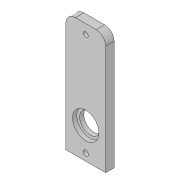
# Autodesk Inventor part: Lidar Sensor Case v4 Piece 1
Saved by Autodesk Inventor 2018.3 (Build 223284000, 284)
## iProperties
Created: 2019-03-27
Part Number: Lidar Sensor Case v4 Piece 1
Material: Generic
Document SubType Name: Modeling
Designer: aye06091
Mass: 10.5036 g
Surface Area: 53.8727 cm^2
Volume: 10.5036 cm^3
Density: 1 g/cm^3
Appearance: Default
Author: aye06091
Autodesk Inventor part; units mm, degrees
ref_plane "YZ Plane" through (0, 0, 0) normal (1, 0, 0) x (0, 1, 0)
ref_plane "XZ Plane" through (0, 0, 0) normal (0, 1, 0) x (-1, 0, 0)
ref_plane "XY Plane" through (0, 0, 0) normal (0, 0, 1) x (1, 0, 0)
sketch "Sketch1" plane through (0, 0, 0) normal (0, 0, 1) x (1, 0, 0)
  line L0 (18.6455, 5.0782) -> (18.6456, 5.0782)
  circle A0 centre (26.2482, -10.4107) radius 8.7948
  line L1 (39.4932, 48.3268) -> (39.4932, -31.0482)
  line L2 (13.0032, -31.0482) -> (13.0032, 48.3268)
  line L3 (13.0032, 48.3268) -> (39.4932, 48.3268)
  line L4 (39.4932, -31.0482) -> (13.0032, -31.0482)
  circle A1 centre (26.2471, -24.96) radius 1.5875
  point P0 (0, 0)
  dimension "d0" = 17.5895
  dimension "d3" = 26.49
  dimension "d4" = 13.245
  dimension "d5" = 58.7375
  dimension "d6" = 79.375
  dimension "d15" = 3.175
  dimension "d25" = 26.49
  dimension "d26" = 13.2461
  constraints: 10 end point, 2 centre point, 2 vertical, 1 horizontal, 1 perpendicular
  measures "d0" diameter of A0
  measures "d3" distance of L2.end L1.start
  measures "d4" distance from line of A0.centre L1
  measures "d5" distance from line of L3 A0.centre
  measures "d6" distance of L1.start L1.end
  measures "d15" diameter of A1
  measures "d25" distance of L1.end L2.start
  measures "d26" distance from line of L1 A1.centre
extrude "Extrusion1" add sketch "Sketch1" against normal blind 5.6134 contours L1 L4 L2 L3 | A1
sketch "Sketch2" plane through (0, 0, 0) normal (0, 0, 1) x (1, 0, 0)
  line L0 (13.0032, 48.3268) -> (39.4932, 48.3268) projected
  circle A0 centre (26.2482, 41.9768) radius 1.6002
  point P0 (0, 0)
  point P1 (0, 0)
  dimension "d10" = 3.2004
  dimension "d12" = 6.35
  constraints: 1 centre point
  measures "d10" diameter of A0
  measures "d12" distance from line of L0 A0.centre
extrude "Extrusion2" cut sketch "Sketch2" against normal blind 5.6134
sketch "Sketch3" plane through (0, 0, 0) normal (0, 0, 1) x (1, 0, 0)
  circle A0 centre (26.2482, -10.4107) radius 8.7947 projected
  circle A1 centre (26.2471, -26.3619) radius 1.7272
  line L0 (39.4932, 48.3268) -> (39.4932, -31.0482) projected
  point P0 (0, 0)
  dimension "d17" = 3.4544
  dimension "d18" = 15.9512
  dimension "d27" = 13.2461
  constraints: 1 centre point
  measures "d17" diameter of A1
  measures "d18" distance of A0.centre A1.centre
  measures "d27" distance from line of L0 A1.centre
extrude "Extrusion3" cut sketch "Sketch3" against normal blind 5.6134 contours A1
fillet "Fillet1" radius 6.35 2 edges at (13.0032, 48.3268, -2.8067) (39.4932, 48.3268, -2.8067)
sketch "Sketch5" plane through (0, 0, -5.6134) normal (0, 0, -1) x (-1, 0, 0)
  circle A0 centre (-26.2482, -10.4107) radius 8.7947 projected
  circle A1 centre (-26.2482, -10.4107) radius 6.9215
  point P0 (0, 0)
  dimension "d28" = 13.843
  constraints: 1 centre point, 1 coincident
  measures "d28" diameter of A1
extrude "Extrusion5" add sketch "Sketch5" against normal blind 2.8067
body "Solid1"
